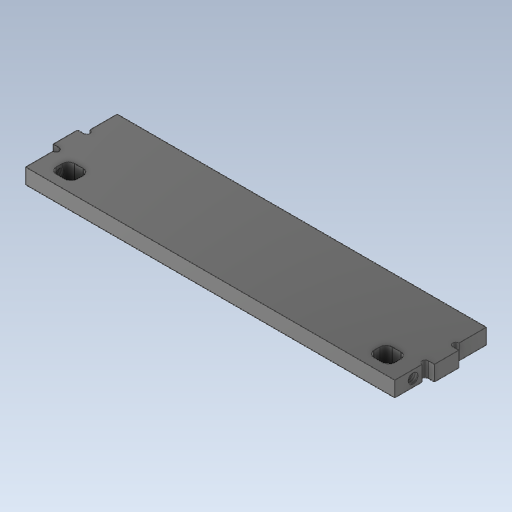
# Autodesk Inventor part: Trunk_back_waisit_frame_
Saved by Autodesk Inventor 2020.4 (Build 244396000, 396)
## iProperties
Created: 2022-01-14
Part Number: Trunk_back_waisit_frame_
Material: アセタール樹脂、黒
Document SubType Name: Modeling
Designer: Masato Kubotera
Density: 1.425 g/cm^3
Appearance: 滑らか - 黒
Description: POM T5
Author: Masato Kubotera
Autodesk Inventor part; units mm, degrees
ref_plane "YZ Plane" through (0, 0, 0) normal (1, 0, 0) x (0, 1, 0)
ref_plane "XZ Plane" through (0, 0, 0) normal (0, 1, 0) x (-1, 0, 0)
ref_plane "XY Plane" through (0, 0, 0) normal (0, 0, 1) x (1, 0, 0)
sketch "スケッチ1" plane through (0, 0, 0) normal (0, 0, 1) x (1, 0, 0)
  line L0 (15, 60.5) -> (-15, 60.5) construction
  line L1 (-15, 60.5) -> (-15, -60.5)
  line L2 (-15, -60.5) -> (15, -60.5)
  line L3 (15, -60.5) -> (15, 60.5)
  line L4 (15, 60.5) -> (-15, -60.5) construction
  line L5 (-15, 60.5) -> (15, -60.5) construction
  line L6 (4, 60.5) -> (4, 62.5)
  line L7 (4, 62.5) -> (-4, 62.5)
  arc A0 (4, 60.5) -> (6.1, 60.5) centre (5.05, 60.5) ccw
  line L8 (0, 62.5) -> (0, 60.5) construction
  line L9 (-4, 60.5) -> (-4, 62.5)
  arc A1 (-6.1, 60.5) -> (-4, 60.5) centre (-5.05, 60.5) ccw
  line L10 (0, 60.5) -> (0, -60.5) construction
  line L11 (15, 0) -> (-15, 0)
  line L12 (-9, 60.5) -> (-9, 55.5) construction
  line L13 (-11, 60.5) -> (-11, 55.5) construction
  line L14 (-7, 60.5) -> (-7, 55.5) construction
  line L15 (11.6254, -55.5) -> (-12, -55.5) construction
  line L16 (-12, -55.5) -> (-12, 55.5) construction
  line L17 (-12, 55.5) -> (11.6254, 55.5) construction
  line L18 (11.6254, 55.5) -> (11.6254, -55.5) construction
  line L19 (11.6254, -55.5) -> (-12, 55.5) construction
  line L20 (-12, -55.5) -> (11.6254, 55.5) construction
  line L21 (-8, 55.5) -> (-10, 55.5)
  line L22 (-12, 53.5) -> (-12, 50.6397)
  line L23 (-10, 48.6397) -> (-8, 48.6397)
  line L24 (-6, 50.6397) -> (-6, 53.5)
  line L25 (-6, 55.5) -> (-12, 48.6397) construction
  line L26 (-12, 55.5) -> (-6, 48.6397) construction
  arc A2 (-6, 53.5) -> (-8, 55.5) centre (-8, 53.5) ccw
  arc A3 (-10, 55.5) -> (-12, 53.5) centre (-10, 53.5) ccw
  arc A4 (-12, 50.6397) -> (-10, 48.6397) centre (-10, 50.6397) ccw
  arc A5 (-8, 48.6397) -> (-6, 50.6397) centre (-8, 50.6397) ccw
  line L27 (6.1, 60.5) -> (15, 60.5)
  line L28 (-6.1, 60.5) -> (-15, 60.5)
  point P0 (0, 0)
  point P1 (-0.1873, 0)
  point P2 (-9, 52.0698)
  point P3 (-9, 52.0698)
  dimension "d0" = 30
  dimension "d1" = 121
  dimension "d2" = 1.05
  dimension "d3" = 2
  dimension "d4" = 0
  dimension "d5" = 8
  dimension "d6" = 5
  dimension "d7" = 3
  dimension "d8" = 4
  dimension "d9" = 9
  dimension "d10" = 2
  constraints: 56 end point, 12 point on circle, 12 point on line, 11 midpoint, 8 tangent, 6 centre point, 5 parallel, 5 symmetric about line, 5 vertical, 4 horizontal, 3 collinear, 3 equal radius, 3 perpendicular, 11 other
  measures "d0" distance of L2.end L1.end
  measures "d1" distance of L1.end L1.start
  measures "d2" radius of A0
  measures "d3" distance of L6.start L6.end
  measures "d4" distance between parallel lines of L8 L10
  measures "d5" distance of L6.end L7.end
  measures "d6" vertical distance of L1.start L16.end
  measures "d7" horizontal distance of L1.start L16.end
  measures "d8" distance of L13.end L14.end
  measures "d9" distance of L12.start L10.start
  measures "d10" radius of A2
extrude "押し出し1" add sketch "スケッチ1" along normal blind 5 contours L28 A1 L9 L7 L6 A0 L27 L3 L11 L1
sketch "スケッチ2" plane through (-15, 60.5, 0) normal (0, 1, 0) x (1, 0, 0)
  line L0 (0, 0) -> (0, -5) projected
  line L1 (0, -2.5) -> (30, -2.5)
  line L2 (30, 0) -> (30, -5) projected
  line L3 (15, 0) -> (15, -5)
  line L4 (19, -5) -> (11, -5) projected
  point P0 (6, -2.5)
  dimension "d13" = 9
  constraints: 4 end point, 3 midpoint, 1 point on line
  measures "d13" distance from line of point (6, -2.5) L3
hole "穴1" at (-9, 60.5, 2.5) direction (0, -1, 0) diameter 3.242 depth 5 tip angle 118 thread size "M4x0.7" class "6H" standard "ISO Metric profile"
mirror "ミラー1" about plane through (-15, 0, 0) normal (0, -1, 0)
